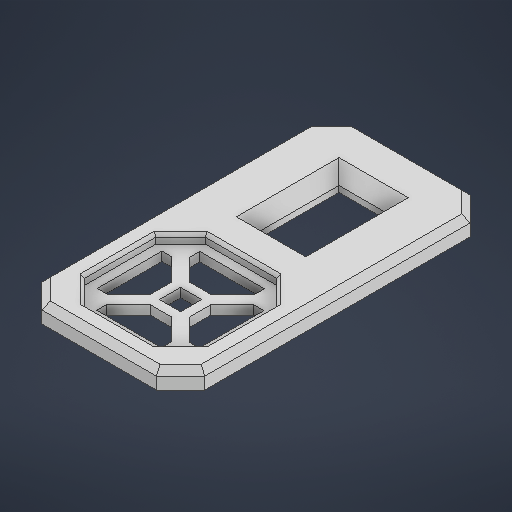
# Autodesk Inventor part: front_pannel_v2
Saved by Autodesk Inventor 2026.2 (Build 302298010, 298A)
## iProperties
Created: 2026-08-06
Part Number: front_pannel_v2
Material: Generic
Document SubType Name: Modeling
Designer: Kugelblitz
Density: 1 g/cm^3
Appearance: Default
Author: Kugelblitz
Autodesk Inventor part; units mm, degrees
ref_plane "YZ Plane" through (0, 0, 0) normal (1, 0, 0) x (0, 1, 0)
ref_plane "XZ Plane" through (0, 0, 0) normal (0, 1, 0) x (-1, 0, 0)
ref_plane "XY Plane" through (0, 0, 0) normal (0, 0, 1) x (1, 0, 0)
sketch "Sketch1" plane through (0, 0, 0) normal (0, 1, 0) x (-1, 0, 0)
  line L0 (-20, 20) -> (20, 20)
  line L1 (20, 20) -> (20, -20)
  line L2 (20, -20) -> (-20, -20)
  line L3 (-20, -20) -> (-20, 20)
  line L4 (-20, 20) -> (20, -20) construction
  line L5 (20, 20) -> (-20, -20) construction
  line L6 (27, 27) -> (-27, 27)
  line L7 (-27, 27) -> (-27, -77)
  line L8 (-27, -77) -> (27, -77)
  line L9 (27, -77) -> (27, 27)
  line L10 (27, -27) -> (-27, -27)
  line L11 (7.5, -39) -> (-7.5, -39)
  line L12 (-7.5, -39) -> (-7.5, -65)
  line L13 (-7.5, -65) -> (7.5, -65)
  line L14 (7.5, -65) -> (7.5, -39)
  line L15 (-27, 19) -> (-19, 27)
  line L16 (27, 19) -> (19, 27)
  line L17 (0, -31.8198) -> (-31.8198, 0)
  line L18 (-31.8198, 0) -> (0, 31.8198)
  line L19 (0, 31.8198) -> (31.8198, 0)
  line L20 (31.8198, 0) -> (0, -31.8198)
  line L21 (0, -31.8198) -> (0, 31.8198) construction
  line L22 (-31.8198, 0) -> (31.8198, 0) construction
  line L23 (-19, -77) -> (-27, -69)
  line L24 (27, -69) -> (19, -77)
  point P0 (0, 0)
  point P1 (20, 0)
  point P2 (0, -27)
  point P3 (0, -65)
  point P4 (-7.5, -52)
  point P5 (-20, -11.8198)
  point P6 (-20, 11.8198)
  point P7 (-11.8198, 20)
  point P8 (11.8198, 20)
  point P9 (20, 11.8198)
  point P10 (20, -11.8198)
  point P11 (11.8198, -20)
  point P12 (-11.8198, -20)
  dimension "d0" = 40
  dimension "d1" = 40
  dimension "d2" = 7
  dimension "d3" = 7
  dimension "d4" = 7
  dimension "d5" = 7
  dimension "d6" = 50
  dimension "d7" = 0
  dimension "d8" = 25
  dimension "d9" = 26
  dimension "d10" = 15
  dimension "d11" = 45
  dimension "d12" = 135
  dimension "d13" = 45
  dimension "d14" = 8
  dimension "d15" = 135
  dimension "d16" = 8
  dimension "d21" = 135
  dimension "d22" = 8
  dimension "d23" = 8
  constraints: 50 end point, 10 point on line, 8 midpoint, 8 parallel, 7 perpendicular, 3 horizontal
  measures "d0" distance of L1.end L2.end
  measures "d1" distance of L0.end L1.end
  measures "d2" distance between parallel lines of L0 L6
  measures "d3" distance from line of point (20, 0) L9
  measures "d4" distance between parallel lines of L7 L3
  measures "d5" distance between parallel lines of L2 L10
  measures "d6" distance between parallel lines of L8 L10
  measures "d7" horizontal distance of point (0, -27) point (0, -65)
  measures "d8" distance from line of L10 point (-7.5, -52)
  measures "d9" distance of L13.end L11.start
  measures "d10" distance of L12.end L13.end
  measures "d11" distance of L17.end L18.end
  measures "d12" angle of L17 L3
  measures "d13" distance of L17.start L17.end
  measures "d14" horizontal distance of L15.start L15.end
  measures "d15" angle of L7 L15
  measures "d16" horizontal distance of L16.start L16.end
  measures "d21" angle of L8 L23
  measures "d22" distance from line of L7 L23.start
  measures "d23" distance of L8.end L24.end
extrude "Extrusion1" add sketch "Sketch1" along normal blind 4 and the other way blind 2 contours L3 L18 L7 L15 L6 L0 | L0 L18 L3 | L18 L6 L19 L0 | L0 L19 L1 L20 L2 L17 L3 L18 | L3 L17 L7 L18 | L19 L6 L16 L9 L1 L0 | L0 L1 L19 | L17 L2 L3 | L3 L2 L17 L10 L7 | L19 L9 L20 L1 | L2 L20 L10 L17 | L20 L9 L10 L2 L1 | L1 L2 L20 | L17 L20 L10 L9 L24 L8 L23 L7 | L10 L20 L17 | L14 L13 L12 L11
sketch "Sketch8" plane through (0, 4, 0) normal (0, 1, 0) x (1, 0, 0)
  line L0 (7.5, 70) -> (7.5, 44) projected
  line L1 (-7.5, 44) -> (-7.5, 70) projected
  line L2 (7.5, 70) -> (-7.5, 70)
  line L3 (-7.5, 70) -> (-7.5, 44)
  line L4 (-7.5, 44) -> (7.5, 44)
  line L5 (7.5, 44) -> (7.5, 70)
  line L6 (-20, 20) -> (20, 20)
  line L7 (20, 20) -> (20, -20)
  line L8 (20, -20) -> (-20, -20)
  line L9 (-20, -20) -> (-20, 20)
  line L10 (20, 11.8198) -> (20, -11.8198) projected
  line L11 (11.8198, -20) -> (-11.8198, -20) projected
  line L12 (-20, -11.8198) -> (-20, 11.8198) projected
  line L13 (-11.8198, 20) -> (11.8198, 20) projected
  line L14 (20, 11.8198) -> (11.8198, 20) projected
  line L15 (20, 11.8198) -> (11.8198, 20)
  line L16 (20, -11.8198) -> (20, 11.8198) projected
  line L17 (20, -11.8198) -> (11.8198, -20) projected
  line L18 (20, -11.8198) -> (11.8198, -20)
  line L19 (-20, -11.8198) -> (-11.8198, -20)
  line L20 (-11.8198, 20) -> (-20, 11.8198)
  point P0 (0, 0)
  point P1 (-11.8198, -20)
  point P2 (11.8198, 20)
  dimension "d35" = 0
  dimension "d36" = 0
  dimension "d37" = 0
  dimension "d38" = 0
  constraints: 24 end point, 6 equal length, 2 horizontal, 2 perpendicular
  measures "d35" distance between parallel lines of L10 L7
  measures "d36" distance between parallel lines of L8 L11
  measures "d37" distance between parallel lines of L9 L12
  measures "d38" distance between parallel lines of L6 L13
extrude "Extrusion3" cut sketch "Sketch8" against normal blind 3 contours L6 L14 L7 L17 L8 L19 L9 L20
sketch "Sketch10" plane through (0, 4, 0) normal (0, 1, 0) x (1, 0, 0)
  line L0 (7.5, 60) -> (-7.5, 60)
  line L1 (-7.5, 60) -> (-7.5, 34)
  line L2 (-7.5, 34) -> (7.5, 34)
  line L3 (7.5, 34) -> (7.5, 60)
  line L4 (19, 77) -> (-19, 77) projected
  point P0 (0, 0)
  point P1 (0, 77)
  point P2 (0, 34)
  point P3 (7.5, 47)
  dimension "d41" = 0
  dimension "d42" = 15
  dimension "d43" = 26
  dimension "d44" = 30
  constraints: 8 end point, 3 midpoint, 2 parallel, 1 horizontal, 1 perpendicular
  measures "d41" horizontal distance of point (0, 77) point (0, 34)
  measures "d42" distance of L0.start L0.end
  measures "d43" distance of L2.end L0.start
  measures "d44" distance from line of point (7.5, 47) L4
extrude "Extrusion4" cut sketch "Sketch10" against normal through all
chamfer "Chamfer1" distance 4 angle 45 4 edges at (7.5, 4, -47) (0, 4, -60) (-7.5, 4, -47) (0, 4, -34)
sketch "Sketch11" plane through (0, 1, 0) normal (0, 1, 0) x (1, 0, 0)
  line L0 (-3.5, 3.5) -> (3.5, 3.5)
  line L1 (3.5, 3.5) -> (3.5, -3.5)
  line L2 (3.5, -3.5) -> (-3.5, -3.5)
  line L3 (-3.5, -3.5) -> (-3.5, 3.5)
  line L4 (-3.5, 3.5) -> (3.5, -3.5) construction
  line L5 (3.5, 3.5) -> (-3.5, -3.5) construction
  line L6 (17, 10.6132) -> (17, -10.818)
  line L7 (20, 11.8198) -> (20, -11.8198) projected
  line L8 (6.5, 3.5) -> (6.5, -3.5)
  line L9 (17, 10.6132) -> (10.2264, 10.6132)
  line L10 (17, -10.818) -> (11.4927, -10.818)
  line L11 (6.5, -3.5) -> (13.818, -10.818)
  line L12 (6.5, 3.5) -> (13.6132, 10.6132)
  line L13 (20, -11.8198) -> (11.8198, -20) projected
  line L14 (11.8198, 20) -> (20, 11.8198) projected
  point P0 (0, 0)
  point P1 (6.5, 0)
  point P2 (3.5, 0)
  dimension "d50" = 7
  dimension "d51" = 7
  dimension "d52" = 3
  dimension "d53" = 3
  dimension "d54" = 0
  dimension "d55" = 7
  constraints: 24 end point, 5 midpoint, 3 horizontal, 3 parallel, 3 perpendicular, 2 vertical, 1 point on line
  measures "d50" distance of L1.end L2.end
  measures "d51" distance of L0.end L1.end
  measures "d52" distance between parallel lines of L6 L7
  measures "d53" distance between parallel lines of L1 L8
  measures "d54" vertical distance of point (6.5, 0) point (3.5, 0)
  measures "d55" distance of L8.start L8.end
extrude "Extrusion5" cut sketch "Sketch11" against normal through all
pattern_circular "Circular Pattern1" count 4 over 360 about axis through (0, -10, 0) along (0, 1, 0) of "Extrusion5"
chamfer "Chamfer2" distance 2 angle 45 8 edges at (-27, 4, -25) (-23, 4, -73) (0, 4, -77) (23, 4, -73) (27, 4, -25) (23, 4, 23) (0, 4, 27) (-23, 4, 23)
chamfer "Chamfer3" distance 1 angle 45 8 edges at (20, 4, 0) (15.9099, 4, -15.9099) (0, 4, -20) (-15.9099, 4, -15.9099) (-20, 4, 0) (-15.9099, 4, 15.9099) (0, 4, 20) (15.9099, 4, 15.9099)
body "Solid1"
